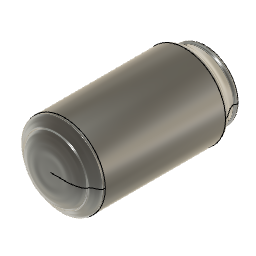
Semana2_DesafioExtra (Autodesk Fusion 360 design; units mm, degrees)
Autodesk Fusion 360 part; units mm, degrees
sketch "Sketch1" plane through (0, 0, 0) normal (0, 0, 1) x (1, 0, 0)
  spline S0 degree 5 poles (-0.0022, 71.9857) (0.1435, 72.0021) (0.4372, 72.0341) (0.8842, 72.08) (1.4933, 72.1366) (2.2763, 72.1998) (3.0804, 72.2554) (3.9047, 72.3035) (4.7475, 72.344) (5.6063, 72.377) (6.4777, 72.4025) (7.3569, 72.4206) (8.2383, 72.4313) (9.1163, 72.4349) (9.9854, 72.4312) (10.841, 72.4204) (11.6798, 72.4025) (12.5006, 72.3774) (13.3044, 72.345) (14.0953, 72.3052) (14.8789, 72.2577) (15.6615, 72.2021) (16.4488, 72.1382) (17.2451, 72.0652) (18.0521, 71.9827) (18.8679, 71.8899) (19.6858, 71.7858) (20.4965, 71.6698) (21.2894, 71.5411) (22.0545, 71.3994) (22.784, 71.2449) (23.4739, 71.0783) (24.1257, 70.9011) (24.7481, 70.7156) (25.353, 70.5244) (25.9519, 70.3299) (26.5523, 70.1337) (27.1542, 69.9359) (27.746, 69.7348) (28.3034, 69.5264) (28.7981, 69.306) (29.2062, 69.0695) (29.5152, 68.8147) (29.7339, 68.5426) (29.8917, 68.2575) (30.0147, 67.9635) (30.1061, 67.661) (30.128, 67.3449) (30.0376, 67.0096) (29.8171, 66.6545) (29.5084, 66.2901) (29.1874, 65.9307) (28.9348, 65.5877) (28.8095, 65.2624) (28.8168, 64.938) (28.9253, 64.5892) (29.0895, 64.1937) (29.274, 63.7462) (29.4621, 63.2598) (29.6485, 62.7562) (29.8354, 62.2589) (30.0281, 61.7853) (30.2302, 61.3384) (30.4438, 60.9105) (30.6699, 60.4893) (30.9095, 60.0632) (31.164, 59.6271) (31.4353, 59.1852) (31.725, 58.7455) (32.033, 58.3162) (32.357, 57.9013) (32.6907, 57.4957) (33.0251, 57.0869) (33.351, 56.6616) (33.6606, 56.2104) (33.9499, 55.7333) (34.2213, 55.2465) (34.4817, 54.7767) (34.7382, 54.3491) (34.9953, 53.9783) (35.2515, 53.6581) (35.4953, 53.3507) (35.7116, 53.0087) (35.8882, 52.5967) (36.0219, 52.1139) (36.1238, 51.6131) (36.1942, 51.2578) (36.2482, 51.0475) (36.2859, 50.9367) (36.3051, 50.8885) knots 0 0 0 0 0 0 0.01176471 0.02352941 0.03529412 0.04705882 0.05882353 0.07058824 0.08235294 0.09411765 0.10588235 0.11764706 0.12941176 0.14117647 0.15294118 0.16470588 0.17647059 0.18823529 0.2 0.21176471 0.22352941 0.23529412 0.24705882 0.25882353 0.27058824 0.28235294 0.29411765 0.30588235 0.31764706 0.32941176 0.34117647 0.35294118 0.36470588 0.37647059 0.38823529 0.4 0.41176471 0.42352941 0.43529412 0.44705882 0.45882353 0.47058824 0.48235294 0.49411765 0.50588235 0.51764706 0.52941176 0.54117647 0.55294118 0.56470588 0.57647059 0.58823529 0.6 0.61176471 0.62352941 0.63529412 0.64705882 0.65882353 0.67058824 0.68235294 0.69411765 0.70588235 0.71764706 0.72941176 0.74117647 0.75294118 0.76470588 0.77647059 0.78823529 0.8 0.81176471 0.82352941 0.83529412 0.84705882 0.85882353 0.87058824 0.88235294 0.89411765 0.90588235 0.91764706 0.92941176 0.94117647 0.95294118 0.96470588 0.97647059 0.98823529 1 1 1 1 1 1
  line L0 (35.1132, 53.8739) -> (37.4969, 47.9032)
  spline S1 degree 5 poles (36.3051, -55.9007) (36.2629, -55.9304) (36.1879, -55.9956) (36.1039, -56.1097) (36.0392, -56.3088) (36.0063, -56.658) (35.9881, -57.1073) (36.0239, -57.4831) (36.0812, -57.7296) (36.0712, -57.9189) (35.9196, -58.1401) (35.6278, -58.4241) (35.2663, -58.7338) (34.9113, -59.0186) (34.6203, -59.2336) (34.3446, -59.4034) (33.9914, -59.5894) (33.5735, -59.7919) (33.1266, -60.0003) (32.7065, -60.1912) (32.3541, -60.3487) (32.0704, -60.4769) (31.8253, -60.5949) (31.5804, -60.7246) (31.3053, -60.8814) (30.9985, -61.0626) (30.6778, -61.2541) (30.3666, -61.4387) (30.0842, -61.6029) (29.83, -61.7464) (29.5882, -61.8807) (29.3415, -62.0224) (29.082, -62.188) (28.8238, -62.3877) (28.5917, -62.6254) (28.4081, -62.898) (28.2807, -63.1951) (28.1901, -63.4989) (28.1037, -63.7896) (27.9881, -64.0517) (27.8239, -64.2798) (27.616, -64.4831) (27.3806, -64.6763) (27.1369, -64.8731) (26.8947, -65.0769) (26.6515, -65.2802) (26.3986, -65.472) (26.1247, -65.6427) (25.8205, -65.7912) (25.4809, -65.9255) (25.1036, -66.0571) (24.6896, -66.1978) (24.2426, -66.3548) (23.7687, -66.5275) (23.2757, -66.709) (22.7717, -66.8893) (22.2641, -67.0573) (21.7589, -67.2035) (21.2596, -67.3223) (20.7656, -67.4148) (20.2737, -67.4868) (19.7789, -67.5469) (19.275, -67.604) (18.7558, -67.6658) (18.2162, -67.7364) (17.6527, -67.8142) (17.0643, -67.8938) (16.4522, -67.9677) (15.8205, -68.0282) (15.177, -68.0693) (14.5318, -68.088) (13.9011, -68.088) (13.3, -68.0769) (12.7337, -68.0593) (12.2022, -68.0396) (11.7004, -68.0208) (11.2203, -68.0049) (10.7518, -67.9933) (10.2848, -67.9864) (9.8097, -67.9841) (9.3175, -67.9857) (8.8, -67.9904) (8.2496, -67.9969) (7.66, -68.0042) (7.0257, -68.0114) (6.3426, -68.0176) (5.6075, -68.0222) (4.8179, -68.0249) (3.9722, -68.0253) (3.0692, -68.0231) (2.1084, -68.0183) (1.2933, -68.0124) (0.6557, -68.0067) (0.219, -68.0023) (-0.0022, -68) knots 0 0 0 0 0 0 0.01111111 0.02222222 0.03333333 0.04444444 0.05555556 0.06666667 0.07777778 0.08888889 0.1 0.11111111 0.12222222 0.13333333 0.14444444 0.15555556 0.16666667 0.17777778 0.18888889 0.2 0.21111111 0.22222222 0.23333333 0.24444444 0.25555556 0.26666667 0.27777778 0.28888889 0.3 0.31111111 0.32222222 0.33333333 0.34444444 0.35555556 0.36666667 0.37777778 0.38888889 0.4 0.41111111 0.42222222 0.43333333 0.44444444 0.45555556 0.46666667 0.47777778 0.48888889 0.5 0.51111111 0.52222222 0.53333333 0.54444444 0.55555556 0.56666667 0.57777778 0.58888889 0.6 0.61111111 0.62222222 0.63333333 0.64444444 0.65555556 0.66666667 0.67777778 0.68888889 0.7 0.71111111 0.72222222 0.73333333 0.74444444 0.75555556 0.76666667 0.77777778 0.78888889 0.8 0.81111111 0.82222222 0.83333333 0.84444444 0.85555556 0.86666667 0.87777778 0.88888889 0.9 0.91111111 0.92222222 0.93333333 0.94444444 0.95555556 0.96666667 0.97777778 0.98888889 1 1 1 1 1 1
  line L1 (38.998, -54.0005) -> (33.6121, -57.8008)
  line L2 (36, -51) -> (36, -63)
  line L3 (37.5971, -57.2405) -> (31.5971, -61.2405)
  line L4 (19.1947, -68.0229) -> (9.7617, -68.1454)
  line L5 (36.3051, 50.8885) -> (36.3051, -55.9007)
  line L6 (-0.0022, -68) -> (-0.0022, 71.9857)
  spline S2 degree 5 poles (27.7789, 67.7767) (27.796, 67.807) (27.8284, 67.8663) (27.872, 67.9507) (27.9198, 68.0542) (27.9625, 68.1687) (27.989, 68.2687) (28.0009, 68.3555) (28.0012, 68.4308) (27.9946, 68.4979) (27.9871, 68.5607) (27.9852, 68.6236) (27.9943, 68.6901) (28.0178, 68.7623) (28.0558, 68.8401) (28.1058, 68.9214) (28.1641, 69.0029) (28.2269, 69.0807) (28.2915, 69.1508) (28.3572, 69.2098) (28.4252, 69.2549) (28.4972, 69.2844) (28.5749, 69.2974) (28.6591, 69.2943) (28.7489, 69.2767) (28.8423, 69.2472) (28.9365, 69.2087) (29.0286, 69.1643) (29.1162, 69.1165) (29.1976, 69.067) (29.2718, 69.0168) (29.3252, 68.9765) (29.3617, 68.9464) (29.3846, 68.9262) (29.3956, 68.9162) knots 0 0 0 0 0 0 0.033333 0.066667 0.1 0.133333 0.166667 0.2 0.233333 0.266667 0.3 0.333333 0.366667 0.4 0.433333 0.466667 0.5 0.533333 0.566667 0.6 0.633333 0.666667 0.7 0.733333 0.766667 0.8 0.833333 0.866667 0.9 0.933333 0.966667 1 1 1 1 1 1
  spline S3 degree 3 poles (27.7789, 67.0104) (27.7799, 67.0097) (27.7846, 67.0063) (27.787, 67.0045) (27.7959, 66.9979) (27.8008, 66.9941) (27.8009, 66.9941) knots 0.461534 0.461534 0.461534 0.461534 0.462551 0.462551 0.462551 0.466294 0.466294 0.466294 0.466294
  spline S4 degree 3 poles (27.6113, 67.2262) (27.6114, 67.2262) (27.6225, 67.2035) (27.639, 67.1716) knots 0.485533 0.485533 0.485533 0.485533 0.492125 0.492125 0.492125 0.492125
  line L7 (1.5076, -65.5136) -> (-0.0022, -65.5021)
  spline S5 degree 3 poles (25.8108, -62.7309) (25.68, -62.8409) (25.4792, -63.005) (25.3088, -63.1447) (25.2723, -63.1747) (25.2369, -63.2037) (25.2033, -63.2314) (25.0145, -63.387) (24.9721, -63.4183) (24.9074, -63.4528) (24.8624, -63.4768) (24.779, -63.5143) (24.6117, -63.5772) (24.1454, -63.7527) (23.2517, -64.058) (22.4229, -64.3577) (21.7586, -64.5978) (21.1748, -64.7834) (20.6484, -64.8896) (20.032, -65.0139) (19.2885, -65.0801) (18.3771, -65.1952) (17.1779, -65.3467) (15.9365, -65.5442) (14.7467, -65.5782) (13.839, -65.6041) (12.9324, -65.5647) (12.1102, -65.5345) (10.5932, -65.4787) (9.3259, -65.4848) (7.5054, -65.5057) (5.982, -65.5232) (4.0187, -65.5325) (1.5076, -65.5136) knots 0.443064 0.443064 0.443064 0.443064 0.466316 0.466316 0.466316 0.471298 0.471298 0.471298 0.500967 0.500967 0.500967 0.521593 0.521593 0.521593 0.577793 0.577793 0.577793 0.624883 0.624883 0.624883 0.679056 0.679056 0.679056 0.750658 0.750658 0.750658 0.804164 0.804164 0.804164 0.902082 0.902082 0.902082 0.984474 0.984474 0.984474 0.984474
  spline S6 degree 3 poles (33.5006, -56.9428) (33.3703, -57.0466) (33.2607, -57.1268) (33.2096, -57.1609) (33.1329, -57.2119) (33.0287, -57.2717) (32.8082, -57.382) (32.4368, -57.5679) (31.8837, -57.8196) (31.4888, -57.9971) (31.036, -58.2007) (30.6556, -58.3772) (30.2247, -58.6208) (29.7458, -58.8916) (29.2261, -59.2115) (28.8669, -59.4179) (28.5978, -59.5726) (28.3046, -59.7166) (27.8608, -60.0047) (27.4822, -60.2505) (26.9649, -60.6359) (26.5289, -61.2321) (26.103, -61.8144) (25.9093, -62.4124) (25.8113, -62.7293) (25.8112, -62.7298) (25.811, -62.7303) (25.8108, -62.7309) knots 0.117918 0.117918 0.117918 0.117918 0.134444 0.134444 0.134444 0.156957 0.156957 0.156957 0.195248 0.195248 0.195248 0.238253 0.238253 0.238253 0.288014 0.288014 0.288014 0.327305 0.327305 0.327305 0.358731 0.358731 0.358731 0.387856 0.387856 0.387856 0.387914 0.387914 0.387914 0.387914
  spline S7 degree 3 poles (33.8071, -55.1679) (33.7894, -55.2095) (33.773, -55.2505) (33.7577, -55.291) (33.5354, -55.8788) (33.5207, -56.3778) (33.5074, -56.6758) (33.5035, -56.7624) (33.5012, -56.8519) (33.5006, -56.9428) knots 0.014528 0.014528 0.014528 0.014528 0.015792 0.015792 0.015792 0.036285 0.036285 0.036285 0.040956 0.040956 0.040956 0.040956
  line L8 (33.8071, 50.5408) -> (33.8071, -55.1679)
  spline S8 degree 3 poles (27.0991, 67.3224) (26.9052, 67.0624) (26.6879, 66.7158) (26.5303, 66.2786) (26.3017, 65.6448) (26.2836, 65.0292) (26.3882, 64.4655) (26.5173, 63.7691) (26.7514, 63.3244) (26.8598, 63.0586) (27.0678, 62.5483) (27.2929, 61.9086) (27.5676, 61.2235) (27.8815, 60.4409) (28.2402, 59.7318) (28.6124, 59.0694) (28.9793, 58.4163) (29.4118, 57.6928) (29.9345, 56.9785) (30.3971, 56.3462) (30.8588, 55.822) (31.1825, 55.3976) (31.4901, 54.9943) (31.7495, 54.5653) (32.0654, 54.0011) (32.3478, 53.4966) (32.6818, 52.9282) (33.044, 52.447) (33.2843, 52.1277) (33.4596, 51.9025) (33.4657, 51.8928) (33.504, 51.8316) (33.5037, 51.8448) (33.5558, 51.657) (33.5598, 51.6425) (33.564, 51.627) (33.5684, 51.6106) (33.6212, 51.4105) (33.687, 51.0355) (33.7867, 50.6229) (33.7932, 50.5961) (33.8, 50.5688) (33.8071, 50.5408) knots 0.580474 0.580474 0.580474 0.580474 0.594639 0.594639 0.594639 0.612787 0.612787 0.612787 0.640673 0.640673 0.640673 0.685524 0.685524 0.685524 0.735313 0.735313 0.735313 0.785034 0.785034 0.785034 0.828797 0.828797 0.828797 0.871792 0.871792 0.871792 0.907955 0.907955 0.907955 0.934418 0.934418 0.934418 0.959854 0.959854 0.959854 0.961814 0.961814 0.961814 0.988549 0.988549 0.988549 0.990238 0.990238 0.990238 0.990238
  line L9 (27.7789, 67.7767) -> (-0.0022, 67.7767)
  line L10 (27.0991, 67.3224) -> (-0.0022, 67.3224)
  point P0 (0, 73)
  point P1 (5.7627, 72.3942)
  point P2 (12.3621, 72.3942)
  point P3 (18, 72)
  point P4 (23.4205, 71.1011)
  point P5 (27, 70)
  point P6 (29.3956, 68.9162)
  point P7 (30, 68)
  point P8 (29.9974, 66.9867)
  point P9 (28.9416, 65.5458)
  point P10 (29.0102, 64.3904)
  point P11 (29.8631, 62.1981)
  point P12 (30.8285, 60.2096)
  point P13 (32.1631, 58.1535)
  point P14 (33.7396, 56.0719)
  point P15 (35.8647, 52.6157)
  point P16 (36.3051, 50.8885)
  point P17 (36.3071, 46.1751)
  point P18 (36.3051, -55.9007)
  point P19 (36, -57)
  point P20 (36, -58)
  point P21 (34.5971, -59.2405)
  point P22 (32.6505, -60.2158)
  point P23 (31.5496, -60.7442)
  point P24 (30.2726, -61.4928)
  point P25 (29.325, -62.0366)
  point P26 (28.4231, -62.902)
  point P27 (28, -64)
  point P28 (27.2574, -64.7761)
  point P29 (26.2753, -65.5441)
  point P30 (24.673, -66.2047)
  point P31 (21.7267, -67.2055)
  point P32 (18.7288, -67.6707)
  point P33 (14.4782, -68.0842)
  point P34 (11, -68)
  point P35 (8, -68)
  point P36 (5.7599, 72.3801)
  point P37 (12.3593, 72.3803)
  point P38 (17.9972, 71.9863)
  point P39 (23.4177, 71.0876)
  point P40 (26.9973, 69.9866)
  point P41 (29.3929, 68.9028)
  point P42 (29.9973, 67.9867)
  point P43 (29.9974, 66.9867)
  point P44 (28.9416, 65.5458)
  point P45 (29.0102, 64.3904)
  point P46 (29.8631, 62.1981)
  point P47 (30.8285, 60.2096)
  point P48 (32.1631, 58.1535)
  point P49 (33.7396, 56.0719)
  point P50 (34.9978, 53.9869)
  point P51 (35.8647, 52.6157)
  point P52 (36, -57)
  point P53 (36, -58)
  point P54 (34.5971, -59.2405)
  point P55 (32.6505, -60.2158)
  point P56 (31.5496, -60.7442)
  point P57 (30.2726, -61.4928)
  point P58 (29.325, -62.0366)
  point P59 (28.4231, -62.902)
  point P60 (28, -64)
  point P61 (27.2574, -64.7761)
  point P62 (26.2753, -65.5441)
  point P63 (24.673, -66.2047)
  point P64 (21.7267, -67.2055)
  point P65 (18.7288, -67.6707)
  point P66 (14.4782, -68.0842)
  point P67 (11, -68)
  point P68 (8, -68)
  point P69 (28, 68.4)
  point P70 (28, 68.7)
  point P71 (28.2358, 69.0885)
  point P72 (28.573, 69.2932)
  point P73 (29.0304, 69.162)
  constraint coincident P43 P8
  constraint coincident P44 P9
  constraint coincident P45 P10
  constraint coincident P46 P11
  constraint coincident P47 P12
  constraint coincident P49 P14
  constraint coincident P51 P15
  constraint coincident P16 S0.end
  constraint midpoint P16 L0
  constraint coincident P48 P13
  constraint coincident P18 S1.start
  constraint coincident P52 P19
  constraint coincident P53 P20
  constraint coincident P54 P21
  constraint coincident P55 P22
  constraint coincident P56 P23
  constraint coincident P57 P24
  constraint coincident P58 P25
  constraint coincident P59 P26
  constraint coincident P60 P27
  constraint coincident P61 P28
  constraint coincident P62 P29
  constraint coincident P63 P30
  constraint coincident P64 P31
  constraint coincident P65 P32
  constraint coincident P66 P33
  constraint coincident P67 P34
  constraint coincident P68 P35
  constraint midpoint P18 L1
  constraint midpoint P52 L2
  constraint midpoint P54 L3
  constraint midpoint P66 L4
  constraint vertical L5
  constraint parallel L5 L6
  constraint coincident S0 P73
  constraint coincident P6 S2.end
  constraint coincident L6 L7.end
  constraint perpendicular L6 L9
  constraint coincident L6 L10.end
  constraint perpendicular L6 L10
  constraint coincident L6 L9.end
revolve "Revolve3" add sketch "Sketch1" angle 360 about axis through (-0.0022, -68, 0) along (0, 1, 0) contours S0 L0 S1 L1 L2 L5 L6 S2 L7 S5 S6 S7 L8 S8 L9 L10 | S0 L0 | S1 L1 L2 | S1 L2
sketch "Sketch3" plane through (0, 67.7767, 0) normal (0, 1, 0) x (-1, 0, 0)
  circle A0 centre (0.0022, 0) radius 27.7811
  line L0 (-3, 17) -> (3, 17)
  line L1 (5, 15) -> (5, 8)
  line L2 (-5, 15) -> (-5, 8)
  arc A1 (-5, 8) -> (5, 8) centre (0, 8) ccw
  line L3 (-1.5, 14.5) -> (1.5, 14.5)
  line L4 (2.5, 13.5) -> (2.5, 12.5)
  line L5 (1.5, 11.5) -> (-1.5, 11.5)
  line L6 (-2.5, 12.5) -> (-2.5, 13.5)
  arc A2 (-2.9999, 8) -> (2.9999, 8) centre (0, 8) ccw
  line L7 (-2.9999, 8) -> (-2.9999, 9)
  line L8 (2.9999, 8) -> (2.9999, 9)
  line L9 (1.9999, 10) -> (-1.9999, 10)
  line L10 (-6, 0) -> (6, 0)
  arc A3 (-3, 17) -> (-5, 15) centre (-3, 15) ccw
  arc A4 (5, 15) -> (3, 17) centre (3, 15) ccw
  arc A5 (-1.5, 14.5) -> (-2.5, 13.5) centre (-1.5, 13.5) ccw
  arc A6 (-2.5, 12.5) -> (-1.5, 11.5) centre (-1.5, 12.5) ccw
  arc A7 (1.5, 11.5) -> (2.5, 12.5) centre (1.5, 12.5) ccw
  arc A8 (2.5, 13.5) -> (1.5, 14.5) centre (1.5, 13.5) ccw
  arc A9 (-1.9999, 10) -> (-2.9999, 9) centre (-1.9999, 9) ccw
  arc A10 (2.9999, 9) -> (1.9999, 10) centre (1.9999, 9) ccw
  point P0 (-5, 17)
  point P1 (5, 17)
  point P2 (-2.9999, 10)
  point P3 (2.9999, 10)
  dimension "d8" = -2.0001
  dimension "d9" = 2
  dimension "d10" = 2
  dimension "d11" = 5
  dimension "d12" = 2.5
  dimension "d13" = 2.5
  dimension "d14" = 9
  dimension "d15" = 10
  dimension "d17" = 1.5
  dimension "d20" = 8
  dimension "d21" = 5
  dimension "d25" = 2
  dimension "d26" = 1
  constraint horizontal L0
  constraint perpendicular L0 L1
  constraint perpendicular L0 L2
  constraint tangent L2 A1
  constraint tangent L1 A1
  constraint horizontal L3
  constraint vertical L4
  constraint horizontal L5
  constraint vertical L6
  constraint vertical L7
  constraint tangent A2 L8
  constraint vertical L8
  constraint horizontal L10
  constraint midpoint origin L10
  constraint coincident P0 L0
  constraint coincident P0 L2
  constraint tangent L0 A3
  constraint tangent L2 A3
  constraint coincident P1 L0
  constraint coincident P1 L1
  constraint tangent L0 A4
  constraint tangent L1 A4
  constraint equal A3 A4
  constraint tangent L3 A5
  constraint tangent L6 A5
  constraint tangent L5 A6
  constraint tangent L6 A6
  constraint equal A5 A6
  constraint tangent L4 A7
  constraint tangent L5 A7
  constraint equal A5 A7
  constraint tangent L3 A8
  constraint tangent L4 A8
  constraint equal A5 A8
  constraint coincident P2 L7
  constraint tangent L7 A9
  constraint tangent L9 A9
  constraint equal A5 A9
  constraint coincident P3 L8
  constraint coincident P3 L9
  constraint tangent L8 A10
  constraint tangent L9 A10
  constraint equal A5 A10
  measures "d9" distance of A2.start P2
  measures "d10" distance of A2.end P3
  measures "d11" distance of L4 L6
  measures "d12" distance of L2 L6
  measures "d13" distance of L0 L3
  measures "d14" distance of P0 L2.end
  measures "d15" distance of P0 P1
  measures "d17" distance of L5 L9
  measures "d20" distance of A1.centre L10
  measures "d21" radius of A1
  measures "d25" radius of A3
  measures "d26" radius of A5
extrude "Extrude1" add sketch "Sketch3" along normal blind 1.2 contours L0 L1 L2 A1 A3 A4
fillet "Fillet1" radius 1 6 edges at (0, 68.9767, 3) (-5, 68.9767, 11.5) (-4.4142, 68.9767, 16.4142) (0, 68.9767, 17) (4.4142, 68.9767, 16.4142) (5, 68.9767, 11.5)
fillet "Fillet2" radius 0.53 14 edges at (-2.9999, 68.9767, 8.5) (0, 68.9767, 5.0001) (2.9999, 68.9767, 8.5) (2.707, 68.9767, 9.7071) (0, 68.9767, 10) (-2.707, 68.9767, 9.7071) (0, 68.9767, 14.5) (-2.2071, 68.9767, 14.2071) (-2.5, 68.9767, 13) (-2.2071, 68.9767, 11.7929) (0, 68.9767, 11.5) (2.2071, 68.9767, 11.7929) (2.5, 68.9767, 13) (2.2071, 68.9767, 14.2071)
